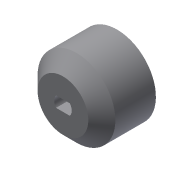
# Autodesk Inventor part: 02_WG_writer_clutch
Saved by Autodesk Inventor 2019.4 (Build 234330000, 330)
## iProperties
Created: 2020-11-13
Part Number: 02_WG_writer_clutch
Material: Generic
Document SubType Name: Modeling
Designer: diederichbenedict
Density: 1 g/cm^3
Appearance: Default
Author: diederichbenedict
Autodesk Inventor part; units mm, degrees
ref_plane "YZ Plane" through (0, 0, 0) normal (1, 0, 0) x (0, 1, 0)
ref_plane "XZ Plane" through (0, 0, 0) normal (0, 1, 0) x (-1, 0, 0)
ref_plane "XY Plane" through (0, 0, 0) normal (0, 0, 1) x (1, 0, 0)
sketch "Sketch1" plane through (0, 0, 0) normal (0, 0, 1) x (1, 0, 0)
  circle A0 centre (0, 0) radius 10 construction
  circle A1 centre (0, 0) radius 11.5
  arc A2 (-3.7696, 9.8) -> (3.7696, 9.8) centre (0, 0) ccw
  line L0 (-3.7696, 9.8) -> (3.7696, 9.8)
  point P0 (0, 0)
  dimension "d0" = 23
  dimension "d1" = 21
  dimension "d2" = 9.8
  constraints: 2 centre point, 2 coincident, 2 end point, 2 point on circle, 1 horizontal
  measures "d0" diameter of A1
  measures "d1" diameter of A2
  measures "d2" distance from line of point (0, 0) L0
extrude "Extrusion1" add sketch "Sketch1" against normal blind 10
pattern_circular "Circular Pattern1" count 3 over 360 about axis through (0, 0, 0) along (0, 0, -1) of "Extrusion1"
sketch "Sketch2" plane through (0, 0, 0) normal (0, 0, 1) x (1, 0, 0)
  circle A0 centre (0, 0) radius 11.5 projected
  line L0 (-3.7696, 9.8) -> (3.7696, 9.8) projected
  arc A1 (10.3719, -1.6354) -> (3.7696, 9.8) centre (0, 0) ccw projected
  line L1 (10.3719, -1.6354) -> (6.6022, -8.1646) projected
  arc A2 (-6.6022, -8.1646) -> (6.6022, -8.1646) centre (0, 0) ccw projected
  line L2 (-6.6022, -8.1646) -> (-10.3719, -1.6354) projected
  arc A3 (-3.7696, 9.8) -> (-10.3719, -1.6354) centre (0, 0) ccw projected
  line L3 (-2, -1.5) -> (2, -1.5) projected
  line L4 (2, 1.5) -> (-2, 1.5) projected
  arc A4 (-2.5, 0) -> (2.5, 0) centre (0, 0) ccw construction
  line L5 (-2.0494, -1.6) -> (2.0494, -1.6)
  line L6 (-2.0494, 1.6) -> (2.0857, 1.6)
  arc A5 (2.0494, -1.6) -> (2.0494, 1.6) centre (0, 0) ccw
  arc A6 (-2.0494, 1.6) -> (-2.0494, -1.6) centre (0, 0) ccw
  point P0 (0, 0)
  dimension "d11" = 0.1
  dimension "d12" = 0.1
  constraints: 4 end point, 4 point on circle, 2 centre point, 1 horizontal, 1 parallel, 1 point on line
  measures "d11" distance between parallel lines of L3 L5
  measures "d12" distance between parallel lines of L4 L6
extrude "Extrusion2" add sketch "Sketch2" along normal blind 6 contours A0 | L0 A1 L1 A2 L2 A3
chamfer "Chamfer1" distance 4 angle 45 1 edges at (-11.5, 0, 6)
body "Solid1"
